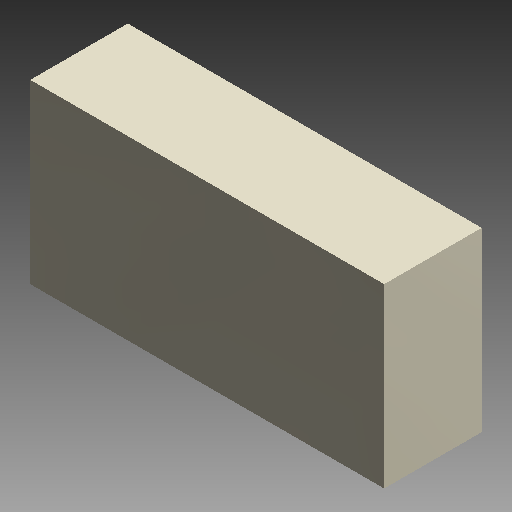
# Autodesk Inventor part: 5988140107F
Saved by Autodesk Inventor 2018.2 (Build 222227000, 227)
## iProperties
Part Number: 5988140107F
Material: Generic
Document SubType Name: Modeling
Designer: autocad
Appearance: LED2012120, 5988140107F
Author: autocad
Autodesk Inventor part; units mm, degrees
ref_plane "YZ Plane" through (0, 0, 0) normal (1, 0, 0) x (0, 1, 0)
ref_plane "XZ Plane" through (0, 0, 0) normal (0, 1, 0) x (-1, 0, 0)
ref_plane "XY Plane" through (0, 0, 0) normal (0, 0, 1) x (1, 0, 0)
sketch "LED2012120, 5988140107F_291" plane through (0, 0, 0) normal (0, 0, 1) x (1, 0, 0)
  line L0 (-1.27, 0.635) -> (1.27, 0.635)
  line L1 (1.27, 0.635) -> (1.27, -0.635)
  line L2 (1.27, -0.635) -> (-1.27, -0.635)
  line L3 (-1.27, -0.635) -> (-1.27, 0.635)
  constraints: 8 end point
extrude "Extrusion1" add sketch "LED2012120, 5988140107F_291" along normal blind 0.7
body "Solid1"
